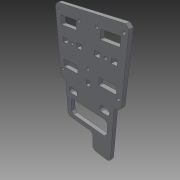
# Autodesk Inventor part: x_carryage_front
Saved by Autodesk Inventor 2014 (Build 180170000, 170)
## iProperties
Created: 2014-03-26
Part Number: x_carryage_front
Material: Generic
Document SubType Name: Modeling
Designer: buben
Density: 1 g/cm^3
Appearance: Default
Mass: 51.3723 g
Surface Area: 201.042 cm^2
Volume: 51.3723 cm^3
Author: buben
Autodesk Inventor part; units mm, degrees
ref_plane "YZ Plane" through (0, 0, 0) normal (1, 0, 0) x (0, 1, 0)
ref_plane "XZ Plane" through (0, 0, 0) normal (0, 1, 0) x (-1, 0, 0)
ref_plane "XY Plane" through (0, 0, 0) normal (0, 0, 1) x (1, 0, 0)
sketch "Sketch1" plane through (0, 0, 0) normal (0, 1, 0) x (-1, 0, 0)
  line L0 (0, 0) -> (-100, 0)
  line L1 (-100, 0) -> (-100, -95.7)
  line L2 (-100, -95.7) -> (0, -95.7)
  line L3 (0, -95.7) -> (0, 0)
  line L4 (-9, -77.5) -> (-32, -77.5)
  line L5 (-33, -76.5) -> (-33, -67.5)
  line L6 (-32, -66.5) -> (-9, -66.5)
  line L7 (-8, -67.5) -> (-8, -76.5)
  arc A0 (-9, -77.5) -> (-8, -76.5) centre (-9, -76.5) ccw
  arc A1 (-33, -76.5) -> (-32, -77.5) centre (-32, -76.5) ccw
  arc A2 (-32, -66.5) -> (-33, -67.5) centre (-32, -67.5) ccw
  arc A3 (-8, -67.5) -> (-9, -66.5) centre (-9, -67.5) ccw
  line L8 (-68, -77.5) -> (-91, -77.5)
  line L9 (-92, -76.5) -> (-92, -67.5)
  line L10 (-91, -66.5) -> (-68, -66.5)
  line L11 (-67, -67.5) -> (-67, -76.5)
  arc A4 (-68, -77.5) -> (-67, -76.5) centre (-68, -76.5) ccw
  arc A5 (-92, -76.5) -> (-91, -77.5) centre (-91, -76.5) ccw
  arc A6 (-91, -66.5) -> (-92, -67.5) centre (-91, -67.5) ccw
  arc A7 (-67, -67.5) -> (-68, -66.5) centre (-68, -67.5) ccw
  line L12 (-9, -23.5) -> (-32, -23.5)
  line L13 (-33, -22.5) -> (-33, -13.5)
  line L14 (-32, -12.5) -> (-9, -12.5)
  line L15 (-8, -13.5) -> (-8, -22.5)
  arc A8 (-9, -23.5) -> (-8, -22.5) centre (-9, -22.5) ccw
  arc A9 (-33, -22.5) -> (-32, -23.5) centre (-32, -22.5) ccw
  arc A10 (-32, -12.5) -> (-33, -13.5) centre (-32, -13.5) ccw
  arc A11 (-8, -13.5) -> (-9, -12.5) centre (-9, -13.5) ccw
  line L16 (-68, -23.5) -> (-91, -23.5)
  line L17 (-92, -22.5) -> (-92, -13.5)
  line L18 (-91, -12.5) -> (-68, -12.5)
  line L19 (-67, -13.5) -> (-67, -22.5)
  arc A12 (-68, -23.5) -> (-67, -22.5) centre (-68, -22.5) ccw
  arc A13 (-92, -22.5) -> (-91, -23.5) centre (-91, -22.5) ccw
  arc A14 (-91, -12.5) -> (-92, -13.5) centre (-91, -13.5) ccw
  arc A15 (-67, -13.5) -> (-68, -12.5) centre (-68, -13.5) ccw
  line L20 (-8, -18) -> (-92, -18) construction
  line L21 (-92, -72) -> (-8, -72) construction
  point P0 (-50, -18)
  point P1 (-50, 0)
  dimension "d0" = 100
  dimension "d1" = 1
  dimension "d2" = 11
  dimension "d3" = 25
  dimension "d4" = 1
  dimension "d5" = 11
  dimension "d6" = 25
  dimension "d7" = 1
  dimension "d8" = 11
  dimension "d9" = 25
  dimension "d10" = 1
  dimension "d11" = 11
  dimension "d12" = 25
  dimension "d13" = 54
  dimension "d14" = 8
  dimension "d15" = 95.7
  dimension "d16" = 18
  constraints: 44 end point, 32 point on circle, 32 tangent, 16 centre point, 12 equal radius, 10 parallel, 6 midpoint, 5 horizontal, 5 perpendicular, 4 collinear, 1 vertical alignment
  measures "d0" distance of L0.start L0.end
  measures "d1" radius of A0
  measures "d2" distance between parallel lines of L6 L4
  measures "d3" distance between parallel lines of L5 L7
  measures "d4" radius of A4
  measures "d5" distance between parallel lines of L10 L8
  measures "d6" distance between parallel lines of L9 L11
  measures "d7" radius of A8
  measures "d8" distance between parallel lines of L14 L12
  measures "d9" distance between parallel lines of L13 L15
  measures "d10" radius of A12
  measures "d11" distance between parallel lines of L18 L16
  measures "d12" distance between parallel lines of L17 L19
  measures "d13" distance of L20.start L21.end
  measures "d14" distance between parallel lines of L1 L9
  measures "d15" distance of L2.end L0.start
  measures "d16" distance from line of L0 L20.start
extrude "Extrusion1" add sketch "Sketch1" along normal blind 6.5
sketch "Sketch2" plane through (0, 6.5, 0) normal (0, 1, 0) x (1, 0, 0)
  line L0 (0, 0) -> (100, 0) projected
  line L1 (100, 0) -> (100, 95.7) projected
  line L2 (0, 95.7) -> (0, 0) projected
  line L3 (0, 44) -> (100, 44) construction
  line L4 (100, 44) -> (100, 37.5) construction
  line L5 (100, 37.5) -> (0, 37.5) construction
  line L6 (0, 37.5) -> (0, 44) construction
  line L7 (9.5, 44) -> (17.5, 44)
  line L8 (17.5, 44) -> (17.5, 37.5)
  line L9 (17.5, 37.5) -> (9.5, 37.5)
  line L10 (9.5, 37.5) -> (9.5, 44)
  line L11 (32.5, 44) -> (40.5, 44)
  line L12 (40.5, 44) -> (40.5, 37.5)
  line L13 (40.5, 37.5) -> (32.5, 37.5)
  line L14 (32.5, 37.5) -> (32.5, 44)
  line L15 (59.5, 44) -> (67.5, 44)
  line L16 (67.5, 44) -> (67.5, 37.5)
  line L17 (67.5, 37.5) -> (59.5, 37.5)
  line L18 (59.5, 37.5) -> (59.5, 44)
  line L19 (82.5, 44) -> (90.5, 44)
  line L20 (90.5, 44) -> (90.5, 37.5)
  line L21 (90.5, 37.5) -> (82.5, 37.5)
  line L22 (82.5, 37.5) -> (82.5, 44)
  line L23 (17.5, 44) -> (32.5, 37.5) construction
  line L24 (32.5, 44) -> (17.5, 37.5) construction
  line L25 (67.5, 44) -> (82.5, 37.5) construction
  line L26 (82.5, 44) -> (67.5, 37.5) construction
  circle A0 centre (25, 40.75) radius 2.25
  circle A1 centre (75, 40.75) radius 2.25
  line L27 (40.5, 40.75) -> (59.5, 40.75) construction
  point P0 (50, 40.75)
  point P1 (50, 0)
  dimension "d19" = 6.5
  dimension "d20" = 37.5
  dimension "d21" = 8
  dimension "d22" = 8
  dimension "d23" = 8
  dimension "d24" = 8
  dimension "d25" = 15
  dimension "d26" = 15
  dimension "d27" = 4.5
  dimension "d28" = 4.5
  dimension "d41" = 50
  constraints: 50 end point, 10 parallel, 8 point on line, 6 midpoint, 5 horizontal, 5 perpendicular, 2 centre point, 2 collinear, 1 vertical alignment
  measures "d19" distance of L5.end L3.start
  measures "d20" distance between parallel lines of L0 L5
  measures "d21" distance between parallel lines of L8 L10
  measures "d22" distance between parallel lines of L12 L14
  measures "d23" distance between parallel lines of L16 L18
  measures "d24" distance between parallel lines of L20 L22
  measures "d25" distance between parallel lines of L14 L8
  measures "d26" distance between parallel lines of L22 L16
  measures "d27" diameter of A0
  measures "d28" diameter of A1
  measures "d41" distance of A1.centre A0.centre
extrude "Extrusion2" cut sketch "Sketch2" against normal through all
sketch "Sketch5" plane through (0, 6.5, 0) normal (0, 1, 0) x (1, 0, 0)
  line L0 (100, 95.7) -> (0, 95.7) projected
  line L1 (0, 95.7) -> (0, 0) projected
  line L2 (9.5, 95.7) -> (9.5, 155.7)
  line L3 (9.5, 155.7) -> (58.5, 155.7)
  line L4 (58.5, 155.7) -> (58.5, 187.7)
  line L5 (58.5, 187.7) -> (90.5, 187.7)
  line L6 (90.5, 187.7) -> (90.5, 95.7)
  line L7 (9.5, 95.7) -> (90.5, 95.7)
  point P0 (50, 95.7)
  point P1 (50, 95.7)
  dimension "d42" = 92
  dimension "d43" = 32
  dimension "d44" = 9.5
  constraints: 12 end point, 4 perpendicular, 3 parallel, 2 midpoint, 2 point on line, 1 coincident
  measures "d42" distance of L5.end L6.end
  measures "d43" distance of L4.end L5.end
  measures "d44" distance between parallel lines of L1 L2
extrude "Extrusion4" add sketch "Sketch5" against normal blind 6.5
sketch "Sketch6" plane through (0, 6.5, 0) normal (0, 1, 0) x (1, 0, 0)
  line L0 (90.5, 95.7) -> (90.5, 187.7) projected
  line L1 (9.5, 155.7) -> (9.5, 95.7) projected
  line L2 (9.5, 95.7) -> (0, 95.7) projected
  line L3 (17.5, 112.7) -> (28.5, 112.7)
  line L4 (30.5, 110.7) -> (30.5, 104.7)
  line L5 (28.5, 102.7) -> (17.5, 102.7)
  line L6 (15.5, 104.7) -> (15.5, 110.7)
  line L7 (17.5, 112.7) -> (15.5, 110.7)
  line L8 (15.5, 104.7) -> (17.5, 102.7)
  line L9 (28.5, 102.7) -> (30.5, 104.7)
  line L10 (28.5, 112.7) -> (30.5, 110.7)
  line L11 (71.5, 112.7) -> (82.5, 112.7)
  line L12 (84.5, 110.7) -> (84.5, 104.7)
  line L13 (82.5, 102.7) -> (71.5, 102.7)
  line L14 (69.5, 104.7) -> (69.5, 110.7)
  line L15 (71.5, 112.7) -> (69.5, 110.7)
  line L16 (69.5, 104.7) -> (71.5, 102.7)
  line L17 (82.5, 102.7) -> (84.5, 104.7)
  line L18 (82.5, 112.7) -> (84.5, 110.7)
  point P0 (15.5, 112.7)
  point P1 (30.5, 102.7)
  point P2 (30.5, 112.7)
  point P3 (15.5, 102.7)
  point P4 (69.5, 112.7)
  point P5 (84.5, 102.7)
  point P6 (84.5, 112.7)
  point P7 (69.5, 102.7)
  point P8 (15.5, 107.7)
  dimension "d47" = 2
  dimension "d48" = 2
  dimension "d49" = 2
  dimension "d50" = 2
  dimension "d51" = 2
  dimension "d52" = 2
  dimension "d53" = 2
  dimension "d54" = 2
  dimension "d55" = 10
  dimension "d56" = 2
  dimension "d57" = 2
  dimension "d58" = 2
  dimension "d59" = 2
  dimension "d60" = 2
  dimension "d61" = 2
  dimension "d62" = 2
  dimension "d63" = 2
  dimension "d64" = 10
  dimension "d65" = 12
  dimension "d66" = 15
  dimension "d67" = 15
  dimension "d68" = 6
  dimension "d69" = 6
  constraints: 32 end point, 16 point on line, 4 parallel, 2 horizontal, 2 perpendicular, 1 collinear, 1 midpoint
  measures "d47" distance of L3.start point (15.5, 112.7)
  measures "d48" distance of L6.end point (15.5, 112.7)
  measures "d49" distance of L6.start point (15.5, 102.7)
  measures "d50" distance of L5.end point (15.5, 102.7)
  measures "d51" distance of L5.start point (30.5, 102.7)
  measures "d52" distance of L4.end point (30.5, 102.7)
  measures "d53" distance of L3.end point (30.5, 112.7)
  measures "d54" distance of L4.start point (30.5, 112.7)
  measures "d55" distance between parallel lines of L5 L3
  measures "d56" distance of L11.start point (69.5, 112.7)
  measures "d57" distance of L14.end point (69.5, 112.7)
  measures "d58" distance of L16.start point (69.5, 102.7)
  measures "d59" distance of L13.end point (69.5, 102.7)
  measures "d60" distance of L17.start point (84.5, 102.7)
  measures "d61" distance of L12.end point (84.5, 102.7)
  measures "d62" distance of L18.start point (84.5, 112.7)
  measures "d63" distance of L12.start point (84.5, 112.7)
  measures "d64" distance between parallel lines of L13 L11
  measures "d65" distance from line of L2 point (15.5, 107.7)
  measures "d66" distance between parallel lines of L4 L6
  measures "d67" distance between parallel lines of L12 L14
  measures "d68" distance between parallel lines of L1 L6
  measures "d69" distance between parallel lines of L0 L12
extrude "Extrusion5" cut sketch "Sketch6" against normal through all
sketch "Sketch7" plane through (0, 6.5, 0) normal (0, 1, 0) x (1, 0, 0)
  line L0 (17.5, 112.7) -> (28.5, 112.7) projected
  line L1 (90.5, 95.7) -> (90.5, 187.7) projected
  line L2 (58.5, 155.7) -> (9.5, 155.7) projected
  line L3 (9.5, 155.7) -> (9.5, 95.7) projected
  line L4 (21.5, 147.7) -> (78.5, 147.7)
  line L5 (82.5, 143.7) -> (82.5, 124.7)
  line L6 (78.5, 120.7) -> (21.5, 120.7)
  line L7 (17.5, 124.7) -> (17.5, 143.7)
  line L8 (21.5, 147.7) -> (17.5, 143.7)
  line L9 (17.5, 124.7) -> (21.5, 120.7)
  line L10 (78.5, 120.7) -> (82.5, 124.7)
  line L11 (82.5, 143.7) -> (78.5, 147.7)
  point P0 (17.5, 147.7)
  point P1 (82.5, 120.7)
  point P2 (82.5, 147.7)
  point P3 (17.5, 120.7)
  dimension "d72" = 4
  dimension "d73" = 4
  dimension "d74" = 4
  dimension "d75" = 4
  dimension "d76" = 4
  dimension "d77" = 4
  dimension "d78" = 4
  dimension "d79" = 4
  dimension "d80" = 8
  dimension "d81" = 8
  dimension "d82" = 8
  dimension "d83" = 8
  constraints: 16 end point, 8 point on line, 2 parallel, 1 horizontal, 1 perpendicular
  measures "d72" distance of L4.start point (17.5, 147.7)
  measures "d73" distance of L7.end point (17.5, 147.7)
  measures "d74" distance of L7.start point (17.5, 120.7)
  measures "d75" distance of L6.end point (17.5, 120.7)
  measures "d76" distance of L6.start point (82.5, 120.7)
  measures "d77" distance of L5.end point (82.5, 120.7)
  measures "d78" distance of L5.start point (82.5, 147.7)
  measures "d79" distance of L4.end point (82.5, 147.7)
  measures "d80" distance between parallel lines of L2 L4
  measures "d81" distance between parallel lines of L3 L7
  measures "d82" distance between parallel lines of L0 L6
  measures "d83" distance between parallel lines of L1 L5
extrude "Extrusion6" cut sketch "Sketch7" against normal through all
chamfer "Chamfer2" distance 4 angle 45 8 edges at (100, 3.25, 0) (0, 3.25, 0) (100, 3.25, -95.7) (90.5, 3.25, -187.7) (58.5, 3.25, -187.7) (58.5, 3.25, -155.7) (9.5, 3.25, -155.7) (0, 3.25, -95.7)
chamfer "Chamfer3" distance 2 angle 45 2 edges at (9.5, 3.25, -95.7) (90.5, 3.25, -95.7)
sketch "Sketch8" plane through (0, 6.5, 0) normal (0, 1, 0) x (1, 0, 0)
  line L0 (4, 0) -> (96, 0) projected
  line L1 (9, 77.5) -> (32, 77.5) projected
  circle A0 centre (37.5, 11.75) radius 2.25
  circle A1 centre (62.5, 11.75) radius 2.25
  line L2 (37.5, 11.75) -> (62.5, 11.75) construction
  point P0 (0, 0)
  point P1 (50, 11.75)
  point P2 (50, 0)
  dimension "d92" = 4.5
  dimension "d93" = 11.75
  dimension "d94" = 25
  constraints: 2 centre point, 2 end point, 2 midpoint, 1 equal radius, 1 horizontal alignment, 1 parallel, 1 vertical alignment
  measures "d92" diameter of A0
  measures "d93" distance from line of L0 L2.start
  measures "d94" distance of L2.start L2.end
extrude "Extrusion7" cut sketch "Sketch8" against normal through all
sketch "Sketch10" plane through (0, 6.5, 0) normal (0, 1, 0) x (1, 0, 0)
  line L0 (0, 91.7) -> (0, 4) projected
  line L1 (4, 0) -> (96, 0) projected
  line L2 (100, 4) -> (100, 91.7) projected
  line L3 (32, 12.5) -> (9, 12.5) projected
  line L4 (8, 67.5) -> (8, 76.5) projected
  line L5 (9, 77.5) -> (32, 77.5) projected
  line L6 (5, 81.75) -> (95, 81.75) construction
  line L7 (95, 81.75) -> (95, 8.25) construction
  line L8 (95, 8.25) -> (5, 8.25) construction
  line L9 (5, 8.25) -> (5, 81.75) construction
  circle A0 centre (5, 81.75) radius 4.5 construction
  circle A1 centre (95, 81.75) radius 4.5 construction
  circle A2 centre (95, 8.25) radius 4.5 construction
  circle A3 centre (5, 8.25) radius 4.5 construction
  circle A4 centre (5, 81.75) radius 2.25
  circle A5 centre (95, 81.75) radius 2.25
  circle A6 centre (95, 8.25) radius 2.25
  circle A7 centre (5, 8.25) radius 2.25
  point P0 (0, 0)
  dimension "d102" = 9
  dimension "d103" = 4.5
  dimension "d104" = 8
  dimension "d105" = 5
  dimension "d106" = 5
  dimension "d107" = 12.5
  dimension "d108" = 8.25
  dimension "d110" = 4.25
  constraints: 8 centre point, 8 coincident, 8 end point, 6 equal radius, 2 parallel, 1 horizontal, 1 perpendicular
  measures "d102" diameter of A0
  measures "d103" diameter of A4
  measures "d104" distance between parallel lines of L4 L0
  measures "d105" distance between parallel lines of L9 L0
  measures "d106" distance between parallel lines of L2 L7
  measures "d107" distance between parallel lines of L1 L3
  measures "d108" distance between parallel lines of L1 L8
  measures "d110" distance between parallel lines of L5 L6
extrude "Extrusion9" cut sketch "Sketch10" against normal through all
sketch "Sketch11" plane through (0, 6.5, 0) normal (0, 1, 0) x (1, 0, 0)
  line L0 (4, 0) -> (96, 0) projected
  line L1 (92, 76.5) -> (92, 67.5) projected
  line L2 (8, 67.5) -> (8, 76.5) projected
  line L3 (8, 76) -> (92, 76) construction
  line L4 (8, 68) -> (92, 68) construction
  circle A0 centre (50, 63.75) radius 2.25
  line L5 (46.75, 86.75) -> (53.25, 86.75)
  line L6 (53.25, 86.75) -> (53.25, 78.75)
  line L7 (53.25, 78.75) -> (46.75, 78.75)
  line L8 (46.75, 78.75) -> (46.75, 86.75)
  point P0 (0, 0)
  point P1 (92, 72)
  point P2 (50, 0)
  point P3 (50, 78.75)
  dimension "d113" = 8
  dimension "d114" = 4
  dimension "d115" = 4.5
  dimension "d116" = 4.25
  dimension "d117" = 6.5
  dimension "d118" = 8
  dimension "d119" = 15
  constraints: 12 end point, 4 point on line, 3 midpoint, 3 perpendicular, 2 parallel, 2 vertical alignment, 1 centre point, 1 horizontal
  measures "d113" distance between parallel lines of L4 L3
  measures "d114" distance from line of point (92, 72) L4
  measures "d115" diameter of A0
  measures "d116" distance from line of L4 A0.centre
  measures "d117" distance of L6.end L7.end
  measures "d118" distance of L5.end L6.end
  measures "d119" distance from line of L7 A0.centre
extrude "Extrusion10" cut sketch "Sketch11" against normal through all
equation "\"d22\" = d21"
equation "\"d23\" = d22"
equation "\"d24\" = d23"
equation "\"d48\" = d47"
equation "\"d49\" = d47"
equation "\"d50\" = d49"
equation "\"d51\" = d47"
equation "\"d52\" = d51"
equation "\"d53\" = d47"
equation "\"d54\" = d53"
equation "\"d57\" = d56"
equation "\"d58\" = d56"
equation "\"d59\" = d58"
equation "\"d60\" = d56"
equation "\"d61\" = d60"
equation "\"d62\" = d56"
equation "\"d63\" = d62"
equation "\"d67\" = d66"
equation "\"d69\" = d68"
equation "\"d73\" = d72"
equation "\"d74\" = d72"
equation "\"d75\" = d74"
equation "\"d76\" = d72"
equation "\"d77\" = d76"
equation "\"d78\" = d72"
equation "\"d79\" = d78"
equation "\"d81\" = d80"
equation "\"d82\" = d80"
equation "\"d83\" = d80"
body "Solid1"
